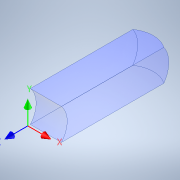
# Autodesk Inventor part: shank_2
Saved by Autodesk Inventor 2020.2 (Build 242310000, 310)
## iProperties
Created: 2021-01-30
Part Number: shank_2
Material: Generic
Document SubType Name: Modeling
Designer: DELL
Density: 1 g/cm^3
Appearance: Clear - Blue
Author: DELL
Autodesk Inventor part; units mm, degrees
ref_plane "YZ Plane" through (0, 0, 0) normal (1, 0, 0) x (0, 1, 0)
ref_plane "XZ Plane" through (0, 0, 0) normal (0, 1, 0) x (-1, 0, 0)
ref_plane "XY Plane" through (0, 0, 0) normal (0, 0, 1) x (1, 0, 0)
sketch "Sketch11" plane through (0, 0, 0) normal (1, 0, 0) x (0, 1, 0)
  line L0 (-2180.7929, 0) -> (12762.7576, 0) construction
  line L1 (0, -333.2) -> (0, 109.2) projected
  circle A0 centre (0, 0) radius 32.5
  circle A1 centre (0, 0) radius 46
  line L2 (-30, -34.8712) -> (-30, -241.9615)
  line L3 (-30, -241.9615) -> (30, -241.9615)
  line L4 (30, -241.9615) -> (30, -34.8712)
  arc A2 (-30, -241.9615) -> (30, -241.9615) centre (0, -190) ccw
  arc A3 (30, -241.9615) -> (50, -223.1662) centre (0, -190) ccw
  line L5 (0, -270) -> (50, -270)
  line L6 (50, -270) -> (50, -223.1662)
  arc A4 (30, -34.8712) -> (32, -240.7543) centre (10627.9646, -34.8712) ccw
  point P0 (-30, -241.9615)
  point P1 (0, -250)
  point P2 (0, -241.9615)
  point P3 (0, -185.7103)
  point P4 (0, -250)
  point P5 (0, -46)
  dimension "d77" = 65
  dimension "d78" = 92
  dimension "d79" = 60
  dimension "d85" = 20
  dimension "d86" = 20
  dimension "d87" = 60
  dimension "d89" = 32
  dimension "d90" = 250
  constraints: 10 end point, 10 point on circle, 5 centre point, 3 coincident, 3 point on line, 2 perpendicular, 2 vertical, 1 horizontal, 1 tangent, 1 other
  measures "d77" diameter of A0
  measures "d78" diameter of A1
  measures "d79" distance between parallel lines of L4 L2
  measures "d85" distance edge to line of A2 L5
  measures "d86" distance from line of L4 L6.end
  measures "d87" radius of A2
  measures "d89" distance from line of A4.end L1
  measures "d90" distance of point (0, -250) A0.centre
extrude "Extrusion11" add sketch "Sketch11" along normal mid plane 60 contours L1 A1 L4 L3
revolve "Revolution1" add sketch "Sketch11" angle 180 mid plane about axis through (0, 0, -10) along (0, 0, 1) picked at (16.8404, -243.4348) contours L1 L3 A2
revolve "Revolution2" cut sketch "Sketch11" angle 360 about axis through (0, 0, -10) along (0, 0, 1) contours L1 A2 A3 L6 L5
mirror "Mirror1" about plane through (0, 0, 0) normal (0, 1, 0)
fillet "Fillet7" [suppressed]
body "Solid1"
body "Solid5"
